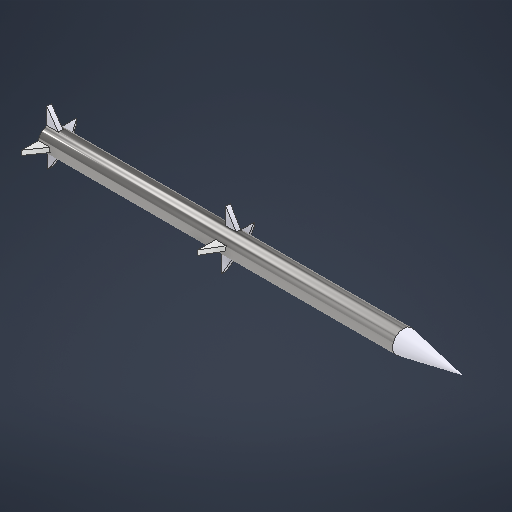
# Autodesk Inventor part: 120c
Saved by Autodesk Inventor 2026.3 (Build 303398000, 398)
## iProperties
Created: 2026-04-13
Part Number: 120c
Material: Genérico
Document SubType Name: Modeling
Designer: warri
Density: 1 g/cm^3
Appearance: Padrão
Author: warri
Autodesk Inventor part; units mm, degrees
ref_plane "YZ Plane" through (0, 0, 0) normal (1, 0, 0) x (0, 1, 0)
ref_plane "XZ Plane" through (0, 0, 0) normal (0, 1, 0) x (-1, 0, 0)
ref_plane "XY Plane" through (0, 0, 0) normal (0, 0, 1) x (1, 0, 0)
sketch "Esboço1" plane through (0, 0, 0) normal (0, 0, 1) x (1, 0, 0)
  line L0 (0, 8.6539) -> (150, 8.6539)
  line L1 (0, 8.6539) -> (0, 0.1539)
  line L2 (150, 8.6539) -> (150, 0.1539)
  line L3 (150, 0.1539) -> (150, 16.6456)
  line L4 (150, 8.6539) -> (270, 8.6539)
  line L5 (270, 8.6539) -> (285, 4.4039)
  line L6 (270, 0.1539) -> (285, 4.4039)
  line L7 (270, 0.1539) -> (0, 0.1539)
  line L8 (270, 8.6539) -> (270, 0.1539)
  dimension "d13" = 150
  dimension "d15" = 120
  dimension "d17" = 17
  constraints: 18 end point, 3 horizontal, 2 vertical, 1 point on line
  measures "d13" distance of L0.start L0.end
  measures "d15" distance of L0.end L4.end
  measures "d17" diameter of L0.start L7
revolve "Revolução1" add sketch "Esboço1" angle 360 about axis through (270, 0.1539, 0) along (-1, 0, 0) contours L0 L2 L7 L1 | L4 L8 L7 L2
sketch "Esboço2" plane through (0, 0, 0) normal (0, 0, 1) x (1, 0, 0)
  line L0 (285, 0.1539) -> (315, 0.1539)
  line L1 (270, 8.6539) -> (270, -8.3461) projected
  line L2 (270, 0.1539) -> (285, 0.1539)
  line L3 (270, 8.6539) -> (270, 0.1539)
  line L4 (315, 0.1539) -> (270, 8.6539)
  point P0 (0, 0)
  constraints: 8 end point, 2 horizontal, 1 midpoint, 1 perpendicular
revolve "Revolução2" add sketch "Esboço2" angle 360 about axis through (285, 0.1539, 0) along (1, 0, 0)
sketch "Esboço3" plane through (0, 0, 0) normal (0, 1, 0) x (-1, 0, 0)
  line L0 (0, 0) -> (-25, 0)
  line L1 (0, -8.5) -> (0, 8.5) projected
  line L2 (0, 0) -> (-50, 0)
  line L3 (-50, 0) -> (-25, 0)
  line L4 (-50, 0) -> (-25, 0)
  line L5 (0, 0) -> (0, 21)
  line L6 (0, 21) -> (-14.7044, 0)
  line L7 (0, 21) -> (26.0415, 21) construction
  dimension "d54" = 21
  dimension "d57" = 125
  constraints: 14 end point, 3 point on line, 2 collinear, 2 horizontal, 1 midpoint
  measures "d54" distance of L5.start L5.end
  measures "d57" angle of L6 L7
sketch "Esboço4" plane through (0, 0, 0) normal (0, 1, 0) x (-1, 0, 0)
  line L0 (-270, -8.5) -> (-270, 8.5) projected
  line L1 (-134.6841, 0) -> (-134.6841, 21.5359)
  line L2 (-134.6841, 21.5359) -> (-147.3807, 0)
  line L3 (-134.6841, 0) -> (-147.3807, 0)
  point P0 (0, 0)
  dimension "d43" = 25
  dimension "d44" = 21.5359
  constraints: 6 end point, 1 horizontal
  measures "d43" distance of L1.end L2.end
  measures "d44" distance of L1.start L1.end
extrude "Extrusão3" add sketch "Esboço4" along normal blind 3.5
pattern_circular "Padrão circular2" count 4 over 360 about axis through (135, 0.1539, 0) along (-1, 0, 0) of "Extrusão3"
sketch "Esboço5" plane through (0, 0.1539, 0) normal (-1, 0, 0) x (0, 0, 1)
  circle A0 centre (0, -0.1539) radius 5
  dimension "d50" = 10
  constraints: 1 centre point, 1 coincident
  measures "d50" diameter of A0
extrude "Extrusão5" add sketch "Esboço3" along normal mid plane 3.5
pattern_circular "Padrão circular3" count 4 over 360 about axis through (135, 0.1539, 0) along (-1, 0, 0) of "Extrusão5"
extrude "Extrusão6" cut sketch "Esboço5" against normal blind 20
